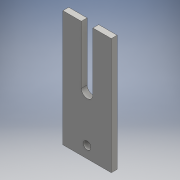
# Autodesk Inventor part: Spacer_lazy_susan
Saved by Autodesk Inventor 2016 (Build 200138000, 138)
## iProperties
Created: 2016-12-13
Part Number: Spacer_lazy_susan
Material: Generic
Document SubType Name: Modeling
Designer: Eivind
Density: 1 g/cm^3
Appearance: Default
Author: Eivind
Autodesk Inventor part; units mm, degrees
ref_plane "YZ Plane" through (0, 0, 0) normal (1, 0, 0) x (0, 1, 0)
ref_plane "XZ Plane" through (0, 0, 0) normal (0, 1, 0) x (-1, 0, 0)
ref_plane "XY Plane" through (0, 0, 0) normal (0, 0, 1) x (1, 0, 0)
sketch "Sketch1" plane through (0, 0, 0) normal (0, 1, 0) x (-1, 0, 0)
  line L0 (0, 0) -> (25, 0)
  line L1 (25, 0) -> (25, -60)
  line L2 (25, -60) -> (0, -60)
  line L3 (0, -60) -> (0, 0)
  point P0 (12.5, -54)
  dimension "d0" = 25
  dimension "d1" = 60
  dimension "d15" = 6
  constraints: 8 end point, 2 parallel, 1 horizontal, 1 perpendicular
  measures "d0" distance of L1.end L2.end
  measures "d1" distance of L0.end L1.end
  measures "d15" distance from line of L2 point (12.5, -54)
extrude "Extrusion1" add sketch "Sketch1" along normal blind 3
sketch "Sketch2" plane through (0, 0, 0) normal (0, -1, 0) x (1, 0, 0)
  point P0 (0, 0)
  point P1 (-12.5, -54)
hole "Hole2" at (-12.5, 0, -54) direction (0, 1, 0) diameter 4 end through all
sketch "Sketch3" plane through (0, 0, 0) normal (0, -1, 0) x (1, 0, 0)
  point P0 (0, 0)
  point P1 (-12.5, -30)
hole "Hole3" at (-12.5, 0, -30) direction (0, 1, 0) diameter 6 end through all
sketch "Sketch4" plane through (0, 0, 0) normal (0, -1, 0) x (1, 0, 0)
  circle A0 centre (-12.5, -30) radius 3 projected
  line L0 (-25, 0) -> (0, 0) projected
  line L1 (-9.5, -30) -> (-15.5, -30)
  line L2 (-15.5, -30) -> (-15.5, 0)
  line L3 (-15.5, 0) -> (-9.5, 0)
  line L4 (-9.5, 0) -> (-9.5, -30)
  constraints: 8 end point, 2 parallel, 1 horizontal, 1 horizontal alignment, 1 perpendicular, 1 point on line, 1 other
extrude "Extrusion2" cut sketch "Sketch4" against normal through all contours L1 A0 | A0 L2 L0 L4 picked at (-11.666, -28.6328)
body "Solid1"
